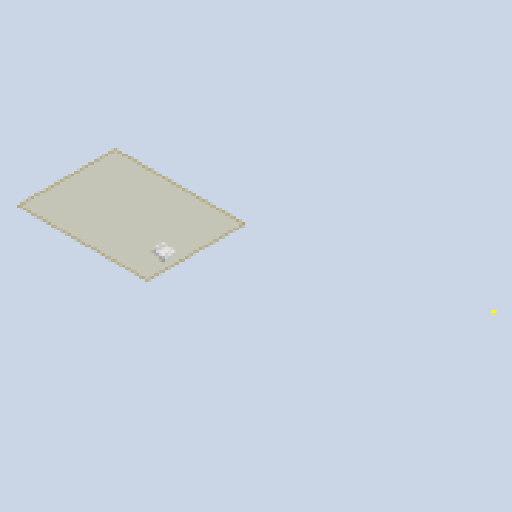
# Autodesk Inventor part: крепление tcrt5000
Saved by Autodesk Inventor 2024.2 (Build 282272000, 272)
## iProperties
Created: 2025-12-05
Part Number: крепление tcrt5000
Material: Типовые
Document SubType Name: Modeling
Designer: katya_notebook
Density: 1 g/cm^3
Appearance: По умолчанию
Author: katya_notebook
Autodesk Inventor part; units mm, degrees
ref_plane "YZ Plane" through (0, 0, 0) normal (1, 0, 0) x (0, 1, 0)
ref_plane "XZ Plane" through (0, 0, 0) normal (0, 1, 0) x (-1, 0, 0)
ref_plane "XY Plane" through (0, 0, 0) normal (0, 0, 1) x (1, 0, 0)
ref_plane "РабПлоскость1" through (-615.1898, 68.3314, 217.435) normal (0, 1, 0) x (-1, 0, 0)
sketch "Эскиз1" plane through (-615.1898, 68.3314, 217.435) normal (0, 1, 0) x (-1, 0, 0)
  circle A0 centre (-129, 47.5) radius 2 projected
  circle A1 centre (-129, 41.5) radius 2 projected
  line L0 (-129, 47.5) -> (-129, 41.5)
  line L1 (-134, 32) -> (-124, 32)
  line L2 (-124, 32) -> (-124, 57)
  line L3 (-124, 57) -> (-134, 57)
  line L4 (-134, 57) -> (-134, 32)
  line L5 (-134, 32) -> (-124, 57) construction
  line L6 (-124, 32) -> (-134, 57) construction
  point P0 (-615.1898, -217.435)
  point P1 (-129, 44.5)
  dimension "d0" = 25
  dimension "d1" = 10
  constraints: 14 end point, 3 midpoint, 2 parallel, 1 horizontal, 1 perpendicular, 1 vertical
  measures "d0" distance of L1.end L2.end
  measures "d1" distance of L1.start L1.end
extrude "Выдавливание1" add sketch "Эскиз1" along normal blind 5
sketch "Эскиз2" plane through (-615.1898, 73.3314, 217.435) normal (0, 1, 0) x (1, 0, 0)
  point P0 (615.1898, 217.435)
sketch "Эскиз3" plane through (-615.1898, 73.3314, 217.435) normal (0, 1, 0) x (1, 0, 0)
  point P0 (615.1898, 217.435)
sketch "Эскиз4" plane through (-615.1898, 73.3314, 217.435) normal (0, 1, 0) x (1, 0, 0)
  line L0 (134, -32) -> (124, -32) projected
  line L1 (134, -32) -> (103.9044, -32)
  line L2 (103.9044, -32) -> (103.9044, -57)
  line L3 (103.9044, -57) -> (134, -57)
  line L4 (134, -57) -> (134, -32)
  circle A0 centre (110.5, -44.5) radius 1.5 projected
  point P0 (615.1898, 217.435)
  constraints: 8 end point, 2 parallel, 1 horizontal, 1 perpendicular
extrude "Выдавливание2" add sketch "Эскиз4" along normal blind 5
sketch "Эскиз5" plane through (-615.1898, 78.3314, 217.435) normal (0, 1, 0) x (1, 0, 0)
  line L0 (124, -32) -> (103.9044, -32) projected
  line L1 (103.9044, -57) -> (124, -57) projected
  line L2 (107.9044, -32) -> (112.9044, -32)
  line L3 (112.9044, -32) -> (112.9044, -57)
  line L4 (112.9044, -57) -> (107.9044, -57)
  line L5 (107.9044, -57) -> (107.9044, -32)
  line L6 (103.9044, -32) -> (103.9044, -57) projected
  point P0 (615.1898, 217.435)
  point P1 (107.9044, -57)
  point P2 (112.9044, -32)
  dimension "d6" = 4
  dimension "d7" = 5
  constraints: 8 end point, 2 parallel, 2 point on line, 1 horizontal, 1 perpendicular
  measures "d6" distance between parallel lines of L5 L6
  measures "d7" distance between parallel lines of L5 L3
extrude "Выдавливание3" add sketch "Эскиз5" along normal up to surface (6.7181 mm away) contours L3 L1 L5 L0
sketch "Эскиз6" plane through (-507.2854, 85.0494, 274.435) normal (0, 1, 0) x (1, 0, 0)
  circle A0 centre (2.5956, 12.5) radius 1.5 projected
  point P0 (507.2854, 274.435)
extrude "Выдавливание4" cut sketch "Эскиз6" against normal blind 17
sketch "Эскиз7" plane through (-615.1898, 68.3314, 217.435) normal (0, -1, 0) x (1, 0, 0)
  circle A0 centre (129, 41.5) radius 2
  circle A1 centre (129, 47.5) radius 2
  point P0 (615.1898, -217.435)
  constraints: 2 centre point, 4 other
extrude "Выдавливание5" cut sketch "Эскиз7" against normal blind 14.5
